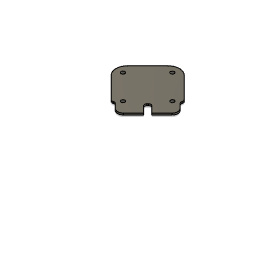
Top (Autodesk Fusion 360 design; units mm, degrees)
Autodesk Fusion 360 part; units mm, degrees
ref_plane "Arbeitsebene1" through (9.1924, 36, 30.4056) normal (0, 1, 0) x (-1, 0, 0)
sketch "Skizze1" plane through (1.0607, 36, 1.0607) normal (0, 1, 0) x (1, 0, 0)
  circle A0 centre (-1.0607, 22.6274) radius 1.6
  circle A1 centre (20.5061, 1.0607) radius 1.6
  circle A2 centre (20.5061, 1.0607) radius 1.6
  circle A3 centre (-22.6274, 1.0607) radius 1.6
  circle A4 centre (-1.0607, 22.6274) radius 1.6
  circle A5 centre (-1.0607, -20.5061) radius 1.6
  arc A6 (1.0607, -29.3449) -> (8.1317, -29.3449) centre (4.5962, -25.8094) ccw
  line L0 (8.1317, -29.3449) -> (29.3449, -8.1317)
  arc A7 (29.3449, -8.1317) -> (29.3449, -1.0607) centre (25.8094, -4.5962) ccw
  line L1 (29.3449, -1.0607) -> (24.0416, 4.2426)
  line L2 (24.0416, 4.2426) -> (25.8094, 6.0104)
  line L3 (25.8094, 6.0104) -> (6.0104, 25.8094)
  arc A8 (6.0104, 25.8094) -> (-8.1317, 25.8094) centre (-1.0607, 18.7383) ccw
  line L4 (-8.1317, 25.8094) -> (-25.8094, 8.1317)
  arc A9 (-25.8094, 8.1317) -> (-25.8094, -6.0104) centre (-18.7383, 1.0607) ccw
  line L5 (-25.8094, -6.0104) -> (-6.0104, -25.8094)
  line L6 (-6.0104, -25.8094) -> (-4.2426, -24.0416)
  line L7 (-4.2426, -24.0416) -> (1.0607, -29.3449)
extrude "Extrusion1" add sketch "Skizze1" along normal blind 1.5
sketch "Skizze2" plane through (0, 37.5, 0) normal (0, 1, 0) x (-1, 0, 0)
  circle A0 centre (0, -21.5668) radius 1.6
  circle A1 centre (0, 21.5668) radius 1.6
  circle A2 centre (-21.5668, 0) radius 1.6
  circle A3 centre (21.5668, 0) radius 1.6
  line L0 (3.182, 25.1023) -> (-2.1213, 30.4056)
  arc A4 (-2.1213, 30.4056) -> (-9.1924, 30.4056) centre (-5.6569, 26.8701) ccw
  line L1 (-9.1924, 30.4056) -> (-30.4056, 9.1924)
  arc A5 (-30.4056, 9.1924) -> (-30.4056, 2.1213) centre (-26.8701, 5.6569) ccw
  line L2 (-30.4056, 2.1213) -> (-25.1023, -3.182)
  line L3 (-25.1023, -3.182) -> (-26.8701, -4.9497)
  line L4 (-26.8701, -4.9497) -> (-7.0711, -24.7487)
  arc A6 (-7.0711, -24.7487) -> (7.0711, -24.7487) centre (0, -17.6777) ccw
  line L5 (7.0711, -24.7487) -> (24.7487, -7.0711)
  arc A7 (24.7487, -7.0711) -> (24.7487, 7.0711) centre (17.6777, 0) ccw
  line L6 (24.7487, 7.0711) -> (4.9497, 26.8701)
  line L7 (4.9497, 26.8701) -> (3.182, 25.1023)
  line L8 (-19.799, 19.799) -> (-12.7279, 12.7279)
  line L9 (-12.7279, 12.7279) -> (-14.4957, 10.9602)
  line L10 (-14.4957, 10.9602) -> (-21.5668, 18.0312)
  line L11 (-12.7279, 12.7279) -> (-10.9602, 14.4957)
  line L12 (-10.9602, 14.4957) -> (-18.0312, 21.5668)
  dimension "d156" = 5
  dimension "d157" = 10
  constraint midpoint L1 L8.start
  constraint perpendicular L1 L8
  constraint perpendicular L8 L9
  constraint coincident L1 L10.end
  constraint perpendicular L1 L10
  constraint perpendicular L8 L11
  constraint coincident L1 L12.end
  constraint perpendicular L1 L12
  constraint equal L9 L11
  measures "d156" distance of L10 L12
  measures "d157" distance of L9.end L10.end
extrude "Extrusion2" cut sketch "Skizze2" against normal blind 2 contours L1 L8 L11 L12 | L1 L8 L9 L10
fillet "Abrundung1" radius 2 6 edges at (26.8701, 36.75, -4.9497) (-4.9497, 36.75, 26.8701) (-3.182, 36.75, 25.1023) (25.1023, 36.75, -3.182) (14.4957, 36.75, 10.9602) (10.9602, 36.75, 14.4957)
sketch "Skizze3" plane through (0, 36, 0) normal (0, -1, 0) x (1, 0, 0)
  arc A0 (-3.9627, 26.0894) -> (-6.1576, 25.6622) centre (-4.7433, 24.248) ccw
  line L0 (-6.1576, 25.6622) -> (-24.7487, 7.0711)
  arc A1 (-24.7487, 7.0711) -> (-24.7487, -7.0711) centre (-17.6777, 0) ccw
  line L1 (-24.7487, -7.0711) -> (-7.0711, -24.7487)
  arc A2 (-7.0711, -24.7487) -> (7.0711, -24.7487) centre (0, -17.6777) ccw
  line L2 (7.0711, -24.7487) -> (25.6622, -6.1576)
  arc A3 (25.6622, -6.1576) -> (26.0894, -3.9627) centre (24.248, -4.7433) ccw
  arc A4 (26.5165, -1.7678) -> (26.0894, -3.9627) centre (27.9307, -3.182) ccw
  line L3 (26.5165, -1.7678) -> (30.4056, 2.1213)
  arc A5 (30.4056, 2.1213) -> (30.4056, 9.1924) centre (26.8701, 5.6569) ccw
  line L4 (30.4056, 9.1924) -> (21.5668, 18.0312)
  line L5 (21.5668, 18.0312) -> (15.9099, 12.3744)
  arc A6 (13.0815, 12.3744) -> (15.9099, 12.3744) centre (14.4957, 13.7886) ccw
  line L6 (13.0815, 12.3744) -> (12.3744, 13.0815)
  arc A7 (12.3744, 15.9099) -> (12.3744, 13.0815) centre (13.7886, 14.4957) ccw
  line L7 (12.3744, 15.9099) -> (18.0312, 21.5668)
  line L8 (18.0312, 21.5668) -> (9.1924, 30.4056)
  arc A8 (9.1924, 30.4056) -> (2.1213, 30.4056) centre (5.6569, 26.8701) ccw
  line L9 (2.1213, 30.4056) -> (-1.7678, 26.5165)
  arc A9 (-3.9627, 26.0894) -> (-1.7678, 26.5165) centre (-3.182, 27.9307) ccw
  circle A10 centre (-21.5668, 0) radius 1.6
  circle A11 centre (21.5668, 0) radius 1.6
  circle A12 centre (0, 21.5668) radius 1.6
  circle A13 centre (0, -21.5668) radius 1.6
  circle A14 centre (0, 21.5668) radius 3
  circle A15 centre (-21.5668, 0) radius 3
  circle A16 centre (0, -21.5668) radius 3
  circle A17 centre (21.5668, 0) radius 3
  dimension "d162" = 6
  dimension "d164" = 360
  constraint concentric A12 A14
  measures "d162" diameter of A14
extrude "Extrusion3" add sketch "Skizze3" along normal blind 1.5 contours A14 | A15 | A16 | A17
fillet "Abrundung2" radius 1.5 4 edges at (-24.3637, 36, 1.0848) (-2.797, 36, 22.6516) (18.7698, 36, 1.0848) (-2.797, 36, -20.4819)
